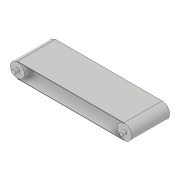
# Autodesk Inventor part: new part ee.2
Saved by Autodesk Inventor 2019 (Build 230136000, 136)
## iProperties
Created: 2019-11-25
Part Number: new part ee.2
Material: Generic
Document SubType Name: Sheet Metal
Designer: Mahesh
Density: 1 g/cm^3
Sheet Metal Rule: Default
Appearance: Default
Author: Mahesh
Autodesk Inventor part; units mm, degrees
ref_plane "YZ Plane" through (0, 0, 0) normal (1, 0, 0) x (0, 1, 0)
ref_plane "XZ Plane" through (0, 0, 0) normal (0, 1, 0) x (-1, 0, 0)
ref_plane "XY Plane" through (0, 0, 0) normal (0, 0, 1) x (1, 0, 0)
sketch "Sketch1" plane through (0, 0, 0) normal (0, 0, 1) x (1, 0, 0)
  arc A0 (201.3738, -100.1974) -> (201.3738, 100.1974) centre (201.3738, 0) ccw
  line L0 (201.3738, 100.1974) -> (201.3738, -100.1974)
  point P0 (0, 0)
  constraints: 2 end point, 2 point on circle, 1 centre point, 1 vertical
extrude "Extrusion1" add sketch "Sketch1" along normal blind 500
sketch "Sketch2" plane through (0, 0, 0) normal (0, 0, -1) x (-1, 0, 0)
  arc A0 (-201.3738, 100.1974) -> (-201.3738, -100.1974) centre (-201.3738, 0) ccw projected
  line L0 (-201.3738, 100.1974) -> (1198.6262, 100.1974)
  line L1 (1198.6262, 100.1974) -> (1198.6262, 95.1974)
  line L2 (1198.6262, 95.1974) -> (-201.3738, 95.1974)
  line L3 (-201.3738, 95.1974) -> (-201.3738, 100.1974)
  line L4 (-201.3738, -100.1974) -> (1198.6262, -100.1974)
  line L5 (1198.6262, -100.1974) -> (1198.6262, -93.0586)
  line L6 (1198.6262, -93.0586) -> (-201.3738, -93.0586)
  line L7 (-201.3738, -93.0586) -> (-201.3738, -100.1974)
  circle A1 centre (-201.3738, 0) radius 93.8222
  point P0 (0, 0)
  dimension "d2" = 1400
  dimension "d3" = 5
  dimension "d4" = 1400
  constraints: 16 end point, 4 parallel, 2 horizontal, 2 perpendicular, 1 centre point, 1 coincident
  measures "d2" distance of L1.end L2.end
  measures "d3" distance of L0.end L1.end
  measures "d4" distance of L6.end L5.end
extrude "Extrusion2" add sketch "Sketch2" against normal blind 500 contours L0 L1 L2 L3
sketch "Sketch3" plane through (0, 0, 0) normal (0, 0, -1) x (-1, 0, 0)
  point P0 (0, 0)
sketch "Sketch4" plane through (0, 0, 0) normal (0, 0, -1) x (-1, 0, 0)
  arc A0 (-201.3738, 100.1974) -> (-201.3738, -100.1974) centre (-201.3738, 0) ccw projected
  line L0 (-201.3738, -100.1974) -> (1198.6262, -100.1974)
  line L1 (1198.6262, -100.1974) -> (1198.6262, -95.1974)
  line L2 (1198.6262, -95.1974) -> (-201.3738, -95.1974)
  line L3 (-201.3738, -95.1974) -> (-201.3738, -100.1974)
  point P0 (0, 0)
  dimension "d7" = 1400
  dimension "d8" = 5
  constraints: 8 end point, 2 parallel, 1 horizontal, 1 perpendicular
  measures "d7" distance of L2.end L1.end
  measures "d8" distance of L1.end L0.end
extrude "Extrusion3" add sketch "Sketch4" against normal blind 500
sketch "Sketch5" plane through (0, 0, 0) normal (0, 0, -1) x (-1, 0, 0)
  line L0 (-201.3738, -95.1974) -> (-201.3738, 95.1974) projected
  circle A0 centre (-201.3738, 0) radius 91.1823
  point P0 (0, 0)
  constraints: 1 centre point, 1 midpoint
extrude "Extrusion4" add sketch "Sketch5" against normal blind 500
sketch "Sketch6" plane through (0, 0, 0) normal (0, 0, -1) x (-1, 0, 0)
  circle A0 centre (1198.807, 0) radius 93.3879
  point P0 (0, 0)
  constraints: 1 centre point
extrude "Extrusion5" add sketch "Sketch6" against normal blind 500
sketch "Sketch7" plane through (-1198.807, 0, 0) normal (0, 0, -1) x (-1, 0, 0)
  circle A0 centre (0, 0) radius 27.7879
  point P0 (-1198.807, 0)
  constraints: 1 centre point
extrude "Extrusion6" add sketch "Sketch7" along normal blind 50
sketch "Sketch8" plane through (-1198.807, 0, 500) normal (0, 0, 1) x (1, 0, 0)
  circle A0 centre (0, 0) radius 27.7879
  point P0 (1198.807, 0)
  constraints: 1 centre point
extrude "Extrusion7" add sketch "Sketch8" along normal blind 50
sketch "Sketch9" plane through (0, 0, 500) normal (0, 0, 1) x (1, 0, 0)
  circle A0 centre (214.5949, 0) radius 24.5251
  point P0 (0, 0)
  constraints: 1 centre point
extrude "Extrusion8" add sketch "Sketch9" along normal blind 50
sketch "Sketch10" plane through (0, 0, 0) normal (0, 0, -1) x (-1, 0, 0)
  circle A0 centre (-210.5074, 0) radius 24.8634
  point P0 (0, 0)
  constraints: 1 centre point
extrude "Extrusion9" add sketch "Sketch10" along normal blind 50
equation "\"BendRadius\" = Thickness"
equation "\"BendReliefWidth\" = Thickness"
equation "\"BendReliefDepth\" = 0.5 * Thickness"
equation "\"CornerReliefSize\" = 4 * Thickness"
equation "\"MinimumRemnant\" = 2 * Thickness"
equation "\"TransitionRadius\" = BendRadius"
equation "\"JacobiRadiusSize\" = BendRadius"
equation "\"GapSize\" = Thickness"
equation "\"Thickness\" = 3.048"
body "Solid1"
